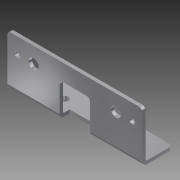
# Autodesk Inventor part: Mounting Bracket V1.500 - (toughbox-mini - sheet metal - underside)
Saved by Autodesk Inventor 2013 (Build 170138000, 138)
## iProperties
Created: 2013-01-13
Part Number: Mounting Bracket V1.500 - (toughbox-mini - sheet metal - underside)
Material: Aluminum 6061-AHC
Document SubType Name: Sheet Metal
Designer: Moses
Density: 2.71 g/cm^3
Flat Pattern Width: 7.14993 cm
Flat Pattern Length: 12.7 cm
Flat Pattern Area: 90.8041 cm^2
Sheet Metal Rule: Default
Sheet Metal Width: 2.815 in
Sheet Metal Length: 5.000 in
Sheet Metal Area: 14.075 in^2
Mass: 66.5965 g
Surface Area: 176.873 cm^2
Volume: 24.5744 cm^3
Author: Moses
Autodesk Inventor part; units mm, degrees
ref_plane "YZ Plane" through (0, 0, 0) normal (1, 0, 0) x (0, 1, 0)
ref_plane "XZ Plane" through (0, 0, 0) normal (0, 1, 0) x (-1, 0, 0)
ref_plane "XY Plane" through (0, 0, 0) normal (0, 0, 1) x (1, 0, 0)
sketch "Sketch1" plane through (0, 0, 0) normal (0, 1, 0) x (-1, 0, 0)
  line L0 (0, 0) -> (127, 0)
  line L1 (127, 0) -> (127, 28.575)
  line L2 (127, 28.575) -> (0, 28.575)
  line L3 (0, 28.575) -> (0, 0)
  dimension "d0" = 127
  dimension "d1" = 28.575
  measures "d0" distance of L0.start L0.end
  measures "d1" distance of L0.end L1.end
extrude "Plate1" add sketch "Sketch1" along normal blind 3.175
sketch "Sketch2" plane through (0, 0, 25.4) normal (0, 0, 1) x (1, 0, 0)
  line L0 (-127, 0) -> (0, 0)
  line L1 (0, 0) -> (0, 47.625)
  line L2 (0, 47.625) -> (-127, 47.625)
  line L3 (-127, 47.625) -> (-127, 0)
  constraints: 6 end point, 1 horizontal, 1 perpendicular, 1 vertical
edge flange "Flange1" height 47.625 angle 90 thickness 3.175 bend radius 1.27 thickness toward (0, 0, 1) relief straight relief width 3.175 relief depth 1.5875 edges at (-63.5, 3.175, 28.575) wall of the first edge with corners at (-127, 0, 25.4) (0, 0, 25.4) (0, 47.625, 25.4) (-127, 47.625, 25.4)
bend "Bend1"
corner "Corner1"
sketch "Sketch3" plane through (-127, 47.625, 28.575) normal (0, 0, 1) x (1, 0, 0)
  line L0 (0, -43.18) -> (127, -43.18) projected
  line L1 (0, 0) -> (127, 0) projected
  line L2 (49.2125, -15.875) -> (77.7875, -15.875)
  line L3 (77.7875, -15.875) -> (77.7875, -47.625)
  line L4 (77.7875, -47.625) -> (49.2125, -47.625)
  line L5 (49.2125, -47.625) -> (49.2125, -15.875)
  line L6 (63.5, 0) -> (63.5, -43.18) construction
  line L7 (127, -47.625) -> (0, -47.625) construction
  point P0 (63.5, -15.875)
  dimension "d18" = 28.575
  dimension "d37" = 31.75
  constraints: 10 end point, 3 midpoint, 2 parallel, 2 point on line, 1 horizontal, 1 perpendicular
  measures "d18" distance of L2.start L2.end
  measures "d37" distance between parallel lines of L7 L2
extrude "Cut1" cut sketch "Sketch3" against normal blind 9.525
sketch "Sketch4" plane through (0, 3.175, 0) normal (0, 1, 0) x (1, 0, 0)
  line L0 (-77.7875, -19.05) -> (-49.2125, -19.05) projected
  line L1 (0, 0) -> (0, -24.13) projected
  line L2 (-127, 0) -> (0, 0) projected
  line L3 (-127, -24.13) -> (-127, 0) projected
  line L4 (-127, -28.575) -> (0, -28.575) projected
  line L5 (-127, -12.7) -> (0, -12.7) construction
  circle A0 centre (-88.9, -12.7) radius 3.302
  circle A1 centre (-38.1, -12.7) radius 3.302
  line L6 (-63.5, -19.05) -> (-63.5, 0) construction
  dimension "d22" = 15.875
  dimension "d23" = 6.604
  dimension "d24" = 6.604
  dimension "d25" = 50.8
  dimension "d26" = 25.4
  constraints: 4 end point, 4 point on line, 2 centre point, 2 midpoint, 1 parallel
  measures "d22" distance between parallel lines of L4 L5
  measures "d23" diameter of A0
  measures "d24" diameter of A1
  measures "d25" distance of A1.centre A0.centre
  measures "d26" distance from line of A1.centre L6
extrude "Cut2" cut sketch "Sketch4" against normal blind 3.175
fillet "Corner Round1" radius 3.175 4 edges at (0, 47.625, 26.9875) (0, 1.5875, 0) (-127, 47.625, 26.9875) (-127, 1.5875, 0)
sketch "Sketch5" plane through (0, 4.445, 25.4) normal (0, 0, -1) x (-1, 0, 0)
  line L0 (111.619, -69.7738) -> (15.381, -69.7738) projected
  arc A0 (111.619, -69.7738) -> (117.9483, -63.937) centre (111.619, -63.4238) ccw projected
  line L1 (127, 47.7012) -> (117.9483, -63.937) projected
  line L2 (127, 49.3522) -> (127, 47.7012) projected
  line L3 (127, 49.3522) -> (0, 49.3522) projected
  line L4 (0, 47.7012) -> (0, 49.3522) projected
  line L5 (9.0517, -63.937) -> (0, 47.7012) projected
  arc A1 (9.0517, -63.937) -> (15.381, -69.7738) centre (15.381, -63.4238) ccw projected
  circle A2 centre (101.092, -60.7835) radius 2.0447 projected
  circle A3 centre (117.475, 28.1165) radius 2.5527 projected
  circle A4 centre (111.125, -60.7835) radius 2.5527 projected
  circle A5 centre (24.765, 28.1165) radius 2.5527 projected
  circle A6 centre (95.25, -60.7835) radius 2.5527 projected
  circle A7 centre (63.5, 9.8044) radius 14.2812 projected
  circle A8 centre (24.765, -18.3655) radius 5.5563 projected
  circle A9 centre (102.235, 7.0345) radius 5.5563 projected
  circle A10 centre (102.235, -18.3655) radius 5.5563 projected
  circle A11 centre (63.5, -30.9118) radius 11.1062 projected
  circle A12 centre (102.235, -43.7655) radius 5.5563 projected
  circle A13 centre (24.765, 7.0345) radius 5.5563 projected
  circle A14 centre (24.765, -43.7655) radius 5.5563 projected
  circle A15 centre (31.75, -60.7835) radius 2.5527 projected
  circle A16 centre (102.235, 28.1165) radius 2.5527 projected
  circle A17 centre (15.875, -60.7835) radius 2.5527 projected
  circle A18 centre (9.525, 28.1165) radius 2.5527 projected
  circle A19 centre (25.908, -60.7835) radius 2.0447 projected
  circle A20 centre (108.077, 28.1165) radius 2.0447 projected
  circle A21 centre (18.923, 28.1165) radius 2.0447 projected
  circle A22 centre (24.765, 28.1165) radius 4.7625
  circle A23 centre (102.235, 28.1165) radius 4.7625
  dimension "d35" = 9.525
  dimension "d36" = 9.525
  constraints: 2 centre point, 2 coincident
  measures "d35" diameter of A22
  measures "d36" diameter of A23
extrude "Cut3" cut sketch "Sketch5" against normal blind 3.175 contours A3 | A5 | A16 | A18 | A23 A20 | A20 A23 | A21 A22 | A21 A22 picked at (106.6712, 28.3745) picked at (105.7103, 29.7674) picked at (20.3435, 28.1165) picked at (21.2688, 29.7707)
sketch "Sketch6" plane through (0, 3.175, 0) normal (0, 1, 0) x (1, 0, 0)
  circle A0 centre (-107.95, -12.7) radius 3.302 projected
  circle A1 centre (-19.05, -12.7) radius 3.302 projected
  point P0 (0, 0)
extrude "Cut4" cut sketch "Sketch6" against normal blind 3.175
fillet "Corner Round2" radius 3.175 2 edges at (-49.2125, 31.75, 26.9875) (-77.7875, 31.75, 26.9875)
equation "\"d24\" = d23"
equation "\"d26\" = 0.5 * d25"
equation "\"d27\" = Thickness"
equation "\"d36\" = d35"
equation "\"d30\" = Thickness"
equation "\"d32\" = Thickness"
equation "\"d4\" = BendReliefWidth"
equation "\"d5\" = BendReliefDepth"
equation "\"d6\" = MinimumRemnant"
equation "\"d7\" = BendRadius"
equation "\"d11\" = CornerReliefSize"
equation "\"d12\" = GapSize"
equation "\"d13\" = JacobiRadiusSize"
equation "\"BendRadius\" = Thickness"
equation "\"BendReliefWidth\" = Thickness"
equation "\"BendReliefDepth\" = 0.5 * Thickness"
equation "\"CornerReliefSize\" = 4 * Thickness"
equation "\"MinimumRemnant\" = 2 * Thickness"
equation "\"TransitionRadius\" = BendRadius"
equation "\"JacobiRadiusSize\" = BendRadius"
equation "\"GapSize\" = Thickness"
equation "\"d3\" = BendRadius"
equation "\"Thickness\" = 3.175"
body "Solid1"
